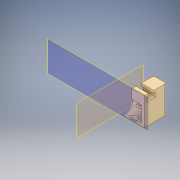
# Autodesk Inventor part: controlBox
Saved by Autodesk Inventor 2017 (Build 210142000, 142)
## iProperties
Created: 2018-08-04
Part Number: controlBox
Material: ABS Plastic
Document SubType Name: Modeling
Designer: Jake
Density: 1.06 g/cm^3
Appearance: Smooth - Off-White
Author: Jake
Autodesk Inventor part; units mm, degrees
ref_plane "YZ Plane" through (0, 0, 0) normal (1, 0, 0) x (0, 1, 0)
ref_plane "XZ Plane" through (0, 0, 0) normal (0, 1, 0) x (-1, 0, 0)
ref_plane "XY Plane" through (0, 0, 0) normal (0, 0, 1) x (1, 0, 0)
sketch "Sketch1" plane through (0, 0, 0) normal (0, 1, 0) x (-1, 0, 0)
  line L0 (70, -46) -> (-70, -46)
  line L1 (-70, -46) -> (-70, 46)
  line L2 (-70, 46) -> (70, 46)
  line L3 (70, 46) -> (70, -46)
  point P0 (0, 0)
  point P1 (0, -46)
  point P2 (-70, 0)
  dimension "d0" = 140
  dimension "d1" = 92
  constraints: 8 end point, 2 midpoint, 2 parallel, 1 horizontal, 1 horizontal alignment, 1 perpendicular, 1 vertical alignment
  measures "d0" distance of L0.start L0.end
  measures "d1" distance of L0.end L1.end
extrude "Extrusion1" add sketch "Sketch1" along normal blind 4
sketch "Sketch2" plane through (0, 4, 0) normal (0, 1, 0) x (1, 0, 0)
  line L0 (70, 46) -> (-70, 46) projected
  line L1 (-70, 46) -> (-70, -46) projected
  line L2 (-70, -46) -> (70, -46) projected
  line L3 (70, -46) -> (70, 46) projected
  line L4 (-70, 46) -> (70, 46)
  line L5 (70, 46) -> (70, -46)
  line L6 (70, -46) -> (-70, -46)
  line L7 (-70, -46) -> (-70, 46)
  line L8 (-66, 42) -> (66, 42)
  line L9 (66, 42) -> (66, -42)
  line L10 (66, -42) -> (-66, -42)
  line L11 (-66, -42) -> (-66, 42)
  point P0 (0, 0)
  point P1 (0, -42)
  dimension "d4" = 4
  dimension "d5" = 4
  dimension "d6" = 4
  dimension "d7" = 4
  constraints: 16 end point, 4 parallel, 2 horizontal, 2 perpendicular, 1 midpoint
  measures "d4" distance between parallel lines of L0 L8
  measures "d5" distance between parallel lines of L1 L11
  measures "d6" distance between parallel lines of L2 L10
  measures "d7" distance between parallel lines of L3 L9
extrude "Extrusion3" add sketch "Sketch2" along normal blind 38.1
sketch "Sketch3" plane through (0, 42.1, 0) normal (0, 1, 0) x (1, 0, 0)
  line L0 (66, 42) -> (66, -42) projected
  line L1 (66, -42) -> (-66, -42) projected
  line L2 (-66, -42) -> (-66, 42) projected
  line L3 (-66, 42) -> (66, 42) projected
  line L4 (70, 46) -> (-70, 46) projected
  line L5 (-70, 46) -> (-70, -46) projected
  line L6 (-70, -46) -> (70, -46) projected
  line L7 (70, -46) -> (70, 46) projected
  line L8 (-66, 42) -> (-66, -42) projected
  line L9 (-66, -42) -> (66, -42) projected
  line L10 (-66, 42) -> (-51, 42)
  line L11 (-51, 42) -> (-51, -42)
  line L12 (-51, -42) -> (-66, -42)
  line L13 (-66, -42) -> (-66, 42)
  line L14 (66, 42) -> (51, 42)
  line L15 (51, 42) -> (51, -42)
  line L16 (51, -42) -> (66, -42)
  line L17 (66, -42) -> (66, 42)
  point P0 (0, 0)
  dimension "d17" = 19
  dimension "d60" = 19
  constraints: 16 end point, 4 parallel, 2 horizontal, 2 perpendicular, 2 point on line
  measures "d17" distance between parallel lines of L5 L11
  measures "d60" distance between parallel lines of L15 L7
extrude "Extrusion4" add sketch "Sketch3" against normal blind 14 contours L0 L1 L15 L3 | L11 L1 L2 L3
sketch "Sketch5" plane through (70, 0, 46) normal (1, 0, 0) x (0, 0, -1)
  line L0 (92, 0) -> (0, 0) projected
  line L1 (92, 0) -> (92, 42.1) projected
  line L2 (0, 42.1) -> (92, 42.1) projected
  line L3 (0, 0) -> (0, 42.1) projected
  line L4 (92, 42.1) -> (0, 42.1) projected
  line L5 (19.15, 42.1) -> (27.15, 42.1)
  line L6 (27.15, 38.1) -> (30.15, 38.1)
  line L7 (30.15, 38.1) -> (30.15, 32.1)
  line L8 (30.15, 32.1) -> (16.15, 32.1)
  line L9 (16.15, 32.1) -> (16.15, 38.1)
  line L10 (16.15, 38.1) -> (19.15, 38.1)
  line L11 (19.15, 38.1) -> (19.15, 42.1)
  line L12 (27.15, 42.1) -> (27.15, 38.1)
  line L13 (64.85, 42.1) -> (72.85, 42.1)
  line L14 (72.85, 38.1) -> (75.85, 38.1)
  line L15 (75.85, 38.1) -> (75.85, 32.1)
  line L16 (75.85, 32.1) -> (61.85, 32.1)
  line L17 (61.85, 32.1) -> (61.85, 38.1)
  line L18 (61.85, 38.1) -> (64.85, 38.1)
  line L19 (64.85, 38.1) -> (64.85, 42.1)
  line L20 (72.85, 42.1) -> (72.85, 38.1)
  line L21 (0, 42.1) -> (92, 42.1) projected
  point P0 (46, 0)
  point P1 (23.15, 42.1)
  point P2 (23.15, 32.1)
  point P3 (68.85, 42.1)
  point P4 (68.85, 32.1)
  dimension "d47" = 14
  dimension "d48" = 6
  dimension "d49" = 8
  dimension "d50" = 10
  dimension "d51" = 23.15
  dimension "d52" = 14
  dimension "d53" = 6
  dimension "d54" = 8
  dimension "d56" = 10
  dimension "d57" = 23.15
  constraints: 32 end point, 8 perpendicular, 6 point on line, 4 midpoint, 2 horizontal, 2 vertical, 2 vertical alignment, 1 collinear
  measures "d47" distance of L7.end L8.end
  measures "d48" distance of L6.end L7.end
  measures "d49" distance between parallel lines of L12 L11
  measures "d50" distance between parallel lines of L2 L8
  measures "d51" distance from line of L3 point (23.15, 42.1)
  measures "d52" distance of L15.end L16.end
  measures "d53" distance of L15.start L15.end
  measures "d54" distance between parallel lines of L20 L19
  measures "d56" distance between parallel lines of L16 L13
  measures "d57" distance from line of point (68.85, 42.1) L1
extrude "Extrusion7" cut sketch "Sketch5" against normal blind 19 contours L20 L14 L15 L16 L17 L18 L19 L2 | L2 L12 L6 L7 L8 L9 L10 L11
sketch "Sketch6" plane through (-70, 0, -46) normal (-1, 0, 0) x (0, 0, 1)
  line L0 (92, 0) -> (0, 0) projected
  line L1 (92, 0) -> (92, 42.1) projected
  line L2 (0, 42.1) -> (92, 42.1) projected
  line L3 (0, 0) -> (0, 42.1) projected
  line L4 (64.85, 42.1) -> (72.85, 42.1)
  line L5 (72.85, 38.1) -> (75.85, 38.1)
  line L6 (75.85, 38.1) -> (75.85, 32.1)
  line L7 (75.85, 32.1) -> (61.85, 32.1)
  line L8 (61.85, 32.1) -> (61.85, 38.1)
  line L9 (61.85, 38.1) -> (64.85, 38.1)
  line L10 (64.85, 38.1) -> (64.85, 42.1)
  line L11 (72.85, 42.1) -> (72.85, 38.1)
  line L12 (19.15, 42.1) -> (27.15, 42.1)
  line L13 (27.15, 38.1) -> (30.15, 38.1)
  line L14 (30.15, 38.1) -> (30.15, 32.1)
  line L15 (30.15, 32.1) -> (16.15, 32.1)
  line L16 (16.15, 32.1) -> (16.15, 38.1)
  line L17 (16.15, 38.1) -> (19.15, 38.1)
  line L18 (19.15, 38.1) -> (19.15, 42.1)
  line L19 (27.15, 42.1) -> (27.15, 38.1)
  line L20 (0, 42.1) -> (92, 42.1) projected
  point P0 (46, 0)
  point P1 (68.85, 42.1)
  point P2 (68.85, 32.1)
  point P3 (23.15, 42.1)
  point P4 (23.15, 32.1)
  dimension "d61" = 14
  dimension "d62" = 6
  dimension "d63" = 8
  dimension "d65" = 14
  dimension "d66" = 6
  dimension "d67" = 8
  dimension "d69" = 10
  dimension "d70" = 23.15
  dimension "d71" = 23.15
  dimension "d72" = 10
  constraints: 32 end point, 8 perpendicular, 4 midpoint, 4 point on line, 2 collinear, 2 horizontal, 2 vertical, 2 vertical alignment
  measures "d61" distance of L6.end L7.end
  measures "d62" distance of L6.start L6.end
  measures "d63" distance between parallel lines of L11 L10
  measures "d65" distance of L14.end L15.end
  measures "d66" distance of L14.start L14.end
  measures "d67" distance between parallel lines of L19 L18
  measures "d69" distance between parallel lines of L7 L4
  measures "d70" distance from line of L3 point (23.15, 42.1)
  measures "d71" distance from line of point (68.85, 42.1) L1
  measures "d72" distance between parallel lines of L15 L12
extrude "Extrusion8" cut sketch "Sketch6" against normal blind 19 contours L11 L5 L6 L7 L8 L9 L10 L2 | L2 L19 L13 L14 L15 L16 L17 L18
sketch "Sketch7" plane through (0, 4, 0) normal (0, 1, 0) x (1, 0, 0)
  line L0 (66, -42) -> (66, 42) projected
  line L1 (66, 42) -> (-66, 42) projected
  line L2 (-66, 42) -> (-66, -42) projected
  line L3 (-66, -42) -> (66, -42) projected
  circle A0 centre (-16, 35) radius 3
  circle A1 centre (-16, -14) radius 3
  circle A2 centre (42, 35) radius 3
  circle A3 centre (42, -14) radius 3
  line L4 (-70, 26.85) -> (-51, 26.85) projected
  line L5 (-51, 26.85) -> (-51, 42) projected
  line L6 (-51, 42) -> (51, 42) projected
  line L7 (51, 42) -> (51, 26.85) projected
  line L8 (51, 26.85) -> (70, 26.85) projected
  line L9 (70, 26.85) -> (70, 46) projected
  line L10 (70, 46) -> (-70, 46) projected
  line L11 (-70, 46) -> (-70, 26.85) projected
  point P0 (0, 0)
  dimension "d75" = 6
  dimension "d76" = 6
  dimension "d77" = 49
  dimension "d78" = 58
  dimension "d79" = 6
  dimension "d80" = 6
  dimension "d82" = 7
  dimension "d92" = 35
  constraints: 4 centre point, 2 horizontal alignment, 2 vertical alignment
  measures "d75" diameter of A0
  measures "d76" diameter of A3
  measures "d77" distance of A3.centre A2.centre
  measures "d78" distance of A3.centre A1.centre
  measures "d79" diameter of A2
  measures "d80" diameter of A1
  measures "d82" distance from line of A0.centre L1
  measures "d92" distance from line of A0.centre L5
extrude "Extrusion9" add sketch "Sketch7" along normal blind 6 contours A0 | A1 | A2 | A3
sketch "Sketch8" plane through (-16, 10, -35) normal (0, 1, 0) x (1, 0, 0)
  circle A0 centre (0, 0) radius 3 projected
  circle A1 centre (0, -49) radius 3 projected
  circle A2 centre (58, 0) radius 3 projected
  circle A3 centre (58, -49) radius 3 projected
  circle A4 centre (58, -49) radius 3 projected
  circle A5 centre (0, 0) radius 3 projected
  point P0 (16, -35)
  constraints: 5 coincident
hole "Hole1" at (-16, 10, -35) at (-16, 10, 14) at (42, 10, -35) at (42, 10, 14) direction (0, -1, 0) diameter 2.75 end through all
sketch "Sketch9" plane through (70, 0, -46) normal (0, 0, -1) x (-1, 0, 0)
  line L0 (19, 38.1) -> (19, 42.1) projected
  line L1 (19, 42.1) -> (19, 38.1) projected
  line L2 (19, 38.1) -> (19, 32.1) projected
  line L3 (19, 32.1) -> (19, 38.1) projected
  line L4 (19, 38.1) -> (19, 42.1) projected
  line L5 (19, 28.1) -> (19, 42.1) projected
  line L6 (19, 42.1) -> (19, 28.1) projected
  line L7 (19, 42.1) -> (19, 38.1) projected
  line L8 (19, 38.1) -> (19, 32.1) projected
  line L9 (19, 32.1) -> (19, 38.1) projected
  line L10 (121, 42.1) -> (121, 38.1) projected
  line L11 (121, 38.1) -> (121, 32.1) projected
  line L12 (121, 32.1) -> (121, 38.1) projected
  line L13 (121, 38.1) -> (121, 42.1) projected
  line L14 (121, 28.1) -> (121, 42.1) projected
  line L15 (121, 42.1) -> (121, 28.1) projected
  line L16 (121, 42.1) -> (121, 38.1) projected
  line L17 (121, 38.1) -> (121, 32.1) projected
  line L18 (121, 32.1) -> (121, 38.1) projected
  line L19 (121, 38.1) -> (121, 42.1) projected
  line L20 (19, 42.1) -> (121, 42.1)
  line L21 (121, 42.1) -> (121, 10)
  line L22 (121, 10) -> (19, 10)
  line L23 (19, 10) -> (19, 42.1)
  line L24 (89, 10) -> (83, 10) projected
  point P0 (70, 0)
  constraints: 8 end point, 2 collinear, 2 parallel, 1 horizontal, 1 perpendicular
extrude "Extrusion10" cut sketch "Sketch9" against normal up to surface (4 mm away)
sketch "Sketch10" plane through (0, 0, 0) normal (0, -1, 0) x (1, 0, 0)
  line L0 (44.3813, -32.6187) -> (39.6188, -32.6188)
  line L1 (39.6188, -32.6188) -> (39.6188, -37.3813)
  line L2 (39.6188, -37.3813) -> (44.3813, -37.3813)
  line L3 (44.3813, -37.3813) -> (44.3813, -32.6187)
  circle A0 centre (42, -35) radius 1.375 projected
  circle A1 centre (42, -35) radius 1.375 projected
  circle A2 centre (-16, -35) radius 1.375 projected
  circle A3 centre (-16, 14) radius 1.375 projected
  circle A4 centre (42, 14) radius 1.375 projected
  line L4 (-70, -46) -> (70, -46) projected
  line L5 (70, -46) -> (70, 46) projected
  line L6 (70, 46) -> (-70, 46) projected
  line L7 (-70, 46) -> (-70, -46) projected
  line L8 (-13.6187, -37.3812) -> (-18.3812, -37.3812)
  line L9 (-18.3812, -37.3812) -> (-18.3812, -32.6187)
  line L10 (-18.3812, -32.6187) -> (-13.6187, -32.6188)
  line L11 (-13.6187, -32.6188) -> (-13.6187, -37.3812)
  line L12 (44.3813, 11.6188) -> (39.6188, 11.6188)
  line L13 (39.6188, 11.6188) -> (39.6188, 16.3813)
  line L14 (39.6188, 16.3813) -> (44.3813, 16.3813)
  line L15 (44.3813, 16.3813) -> (44.3813, 11.6188)
  line L16 (-13.6187, 11.6188) -> (-18.3812, 11.6188)
  line L17 (-18.3812, 11.6188) -> (-18.3812, 16.3813)
  line L18 (-18.3812, 16.3813) -> (-13.6187, 16.3813)
  line L19 (-13.6187, 16.3813) -> (-13.6187, 11.6188)
  point P0 (0, 0)
  point P1 (42, -32.6187)
  point P2 (39.6188, -35)
  point P3 (-18.3812, -35)
  point P4 (-18.3812, 14)
  point P5 (39.6188, 14)
  point P6 (-16, -37.3813)
  point P7 (-16, 11.6188)
  point P8 (42, 11.6188)
  dimension "d95" = 4.7625
  dimension "d96" = 4.7625
  dimension "d97" = 4.7625
  dimension "d98" = 4.7625
  dimension "d99" = 4.7625
  dimension "d100" = 4.7625
  dimension "d101" = 4.7625
  dimension "d102" = 4.7625
  constraints: 32 end point, 8 midpoint, 8 parallel, 4 horizontal, 4 horizontal alignment, 4 perpendicular, 4 vertical alignment
  measures "d95" distance of L0.start L0.end
  measures "d96" distance of L0.end L1.end
  measures "d97" distance of L12.start L12.end
  measures "d98" distance of L12.end L13.end
  measures "d99" distance of L8.start L8.end
  measures "d100" distance of L8.end L9.end
  measures "d101" distance of L16.start L16.end
  measures "d102" distance of L16.end L17.end
extrude "Extrusion11" cut sketch "Sketch10" against normal blind 1.5875 contours L3 L2 L1 L0 | L8 L9 L10 L11 | L12 L13 L14 L15 | L16 L17 L18 L19
sketch "Sketch11" plane through (0, 4, 0) normal (0, 1, 0) x (1, 0, 0)
  circle A0 centre (42, 35) radius 3 projected
  circle A1 centre (-16, 35) radius 3 projected
  circle A2 centre (-16, -14) radius 3 projected
  circle A3 centre (42, -14) radius 3 projected
  line L0 (66, -42) -> (66, 42) projected
  line L1 (66, 42) -> (-66, 42) projected
  line L2 (-66, 42) -> (-66, -42) projected
  line L3 (-66, -42) -> (66, -42) projected
  circle A4 centre (30.3953, -27.3279) radius 6.6721
  circle A5 centre (13, 10.5) radius 26.9638
  circle A6 centre (-27.6047, -27.3279) radius 6.6721
  circle A7 centre (-36.1, 10.5) radius 14.1362
  circle A8 centre (-51.3279, -27.3279) radius 6.6721
  circle A9 centre (52.9819, 10.5) radius 5.0181
  circle A10 centre (42, -14) radius 1.375 construction
  circle A11 centre (13, 10.5) radius 37.9638 construction
  circle A12 centre (-36.1, 10.5) radius 31.6901 construction
  point P0 (0, 0)
  point P1 (-66, 0)
  dimension "d105" = 8
  dimension "d106" = 8
  dimension "d107" = 8
  dimension "d108" = 8
  dimension "d109" = 8
  dimension "d110" = 8
  dimension "d112" = 8
  dimension "d113" = 8
  dimension "d114" = 8
  dimension "d115" = 8
  dimension "d116" = 8
  constraints: 8 centre point, 5 point on circle, 4 horizontal alignment, 2 coincident, 1 midpoint
  measures "d106" distance edge to line of A9 L0
  measures "d109" distance edge to line of A4 L3
  measures "d113" distance edge to line of A6 L3
  measures "d114" distance edge to line of A8 L2
  measures "d115" distance edge to line of A8 L3
extrude "Extrusion12" cut sketch "Sketch11" against normal through all contours A4 | A5 | A6 | A7 | A8 | A9
fillet "Fillet1" radius 2 38 edges at (51, 26.05, -46) (70, 21.05, -46) (0, 10, -46) (0, 10, -42) (-51, 26.05, -46) (-70, 21.05, -46) (-70, 21.05, 46) (66, 16.05, 42) (0, 4, 42) (66, 4, 0) (51, 19.05, -42) (51, 35.1, 42) (47.9638, 4, -10.5) (-13.9638, 4, -10.5) (23.7232, 4, 27.3279) (-51, 35.1, 42) (-51, 19.05, -42) (-66, 4, 0) (-66, 16.05, 42) (-66, 16.05, -42) (0, 4, -42) (-50.2362, 4, -10.5) (-58, 4, 27.3279) (-34.2768, 4, 27.3279) (66, 16.05, -42) (39, 4, 14) (-19, 4, 14) (39, 4, -35) (-19, 4, -35) (70, 21.05, 46) (-51, 28.1, 0) (51, 28.1, 0) (66, 28.1, 0) (-66, 28.1, 0) (-58.5, 28.1, 42) (58.5, 28.1, 42) (58.5, 28.1, -42) (-58.5, 28.1, -42)
ref_plane "Work Plane1" through (70, 0, -12.6625) normal (0, 0, -1) x (-1, 0, 0)
ref_plane "Work Plane2" through (30.3125, 0, 46) normal (1, 0, 0) x (0, 0, -1)
sketch "Sketch12" plane through (70, 0, -12.6625) normal (0, 0, -1) x (-1, 0, 0)
  line L0 (-7.5665, 44.2151) -> (155.3884, 44.2151)
  line L1 (155.3884, 44.2151) -> (155.3884, -4.8886)
  line L2 (155.3884, -4.8886) -> (-7.5665, -4.8886)
  line L3 (-7.5665, -4.8886) -> (-7.5665, 44.2151)
  point P0 (70, 0)
  constraints: 8 end point, 2 parallel, 1 horizontal, 1 perpendicular
extrude "Extrusion13" cut sketch "Sketch12" against normal through all
sketch "Sketch13" plane through (30.3125, 0, 46) normal (1, 0, 0) x (0, 0, -1)
  line L0 (110.5301, 56.5997) -> (-15.9229, 56.5997)
  line L1 (-15.9229, 56.5997) -> (-15.9229, -18.7941)
  line L2 (-15.9229, -18.7941) -> (110.5301, -18.7941)
  line L3 (110.5301, -18.7941) -> (110.5301, 56.5997)
  point P0 (46, 0)
  constraints: 8 end point, 2 parallel, 1 horizontal, 1 perpendicular
extrude "Extrusion14" cut sketch "Sketch13" against normal through all
equation "\"d5\" = d4"
equation "\"d6\" = d4"
equation "\"d7\" = d4"
equation "\"d60\" = d17"
equation "\"d56\" = d50"
equation "\"d57\" = d51"
equation "\"d69\" = d72"
equation "\"d71\" = d70"
equation "\"d76\" = d75"
equation "\"d79\" = d75"
equation "\"d80\" = d75"
equation "\"d96\" = d95"
equation "\"d97\" = d95"
equation "\"d98\" = d96"
equation "\"d99\" = d96"
equation "\"d100\" = d96"
equation "\"d101\" = d96"
equation "\"d102\" = d96"
equation "\"d106\" = d105"
equation "\"d107\" = d106"
equation "\"d108\" = d105"
equation "\"d110\" = d108"
equation "\"d112\" = d105"
equation "\"d113\" = d110"
equation "\"d114\" = d112"
equation "\"d115\" = d112"
equation "\"d116\" = d112"
body "Solid1"
